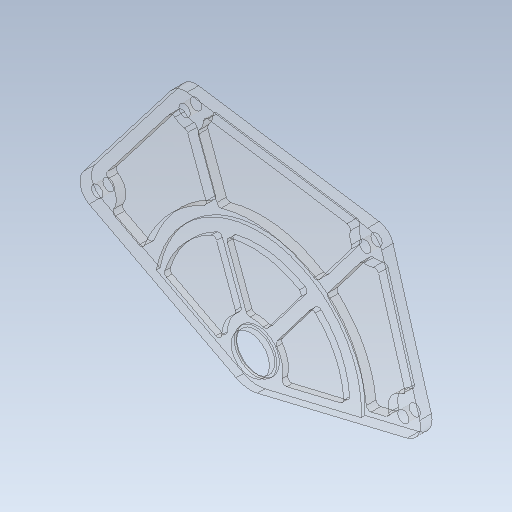
# Autodesk Inventor part: 後ろ脚外フレーム
Saved by Autodesk Inventor 2020 (Build 240168000, 168)
## iProperties
Created: 2019-09-18
Part Number: 後ろ脚外フレーム
Material: ポリカーボネート、クリア
Document SubType Name: Modeling
Designer: tanjihayato
Density: 1.2 g/cm^3
Appearance: ポリカーボネート - クリア
Mass: 5.9648 g
Surface Area: 89.9644 cm^2
Volume: 4.97067 cm^3
Author: tanjihayato
Autodesk Inventor part; units mm, degrees
ref_plane "YZ Plane" through (0, 0, 0) normal (1, 0, 0) x (0, 1, 0)
ref_plane "XZ Plane" through (0, 0, 0) normal (0, 1, 0) x (-1, 0, 0)
ref_plane "XY Plane" through (0, 0, 0) normal (0, 0, 1) x (1, 0, 0)
sketch "スケッチ1" plane through (0, 0, 0) normal (0, 0, 1) x (1, 0, 0)
  circle A0 centre (0, 0) radius 10.1 construction
  circle A1 centre (25.3202, -9.9362) radius 17.1 construction
  circle A2 centre (110.4743, -16.4118) radius 28.1 construction
  circle A3 centre (62.4131, -12.7569) radius 20.1 construction
  circle A4 centre (-21.6908, -16.4118) radius 17.1 construction
  circle A5 centre (-105.5257, -16.4118) radius 28.1 construction
  line L0 (-170.915, -81.4118) -> (490.0044, -81.4118)
  line L1 (-105.5257, -16.4118) -> (-21.6908, -16.4118) construction
  line L2 (110.4743, -16.4118) -> (25.3202, -9.9362) construction
  line L3 (110.4743, -16.4118) -> (104.1501, -0.632)
  line L4 (104.1501, -0.632) -> (95.5937, 20.7173) construction
  line L5 (95.5937, 20.7173) -> (70.4743, -10.4118) construction
  line L6 (70.4743, -10.4118) -> (110.4743, -16.4118) construction
  line L7 (-137.6819, 53.5882) -> (165.8186, 53.5882)
  line L8 (25.3202, -9.9362) -> (108.6869, 8.5882) construction
  line L9 (25.3202, -9.9362) -> (102.5386, -46.4118) construction
  line L10 (25.3202, -9.9362) -> (5.9362, 53.5882) construction
  line L11 (5.9362, 53.5882) -> (127.6431, 30.2622)
  line L12 (127.6431, 30.2622) -> (110.4743, -16.4118) construction
  line L13 (102.5386, -46.4118) -> (118.0681, 0.8329) construction
  line L14 (118.0681, 0.8329) -> (5.9362, 53.5882) construction
  line L15 (108.6869, 8.5882) -> (129.8583, 53.5882) construction
  line L16 (129.8583, 53.5882) -> (5.9362, 53.5882) construction
  line L17 (119.2726, 31.0882) -> (366.4441, 68.5882) construction
  line L18 (119.0587, 6.9252) -> (362.0213, 65.8249) construction
  line L19 (110.3034, -22.7894) -> (351.0624, 44.5537) construction
  line L20 (127.6431, 30.2622) -> (4.1927, 19.4617) construction
  circle A6 centre (80.4743, 23.124) radius 3 construction
  circle A7 centre (80.4743, 23.124) radius 1.5
  arc A8 (79.801, 27.5733) -> (76.162, 24.4099) centre (80.4743, 23.124) ccw
  circle A9 centre (70.4743, -10.4118) radius 1.5
  arc A10 (66.162, -9.1259) -> (69.4242, -14.7876) centre (70.4743, -10.4118) ccw
  circle A11 centre (150.4743, 0.5882) radius 1.5
  arc A12 (152.5623, -3.3981) -> (154.0408, 3.3323) centre (150.4743, 0.5882) ccw
  circle A13 centre (127.6431, 30.2622) radius 1.5
  arc A14 (131.2816, 32.9102) -> (126.9698, 34.7115) centre (127.6431, 30.2622) ccw
  circle A15 centre (110.4743, -16.4118) radius 5
  arc A16 (108.6075, -24.1909) -> (114.1862, -23.4986) centre (110.4743, -16.4118) ccw
  line L21 (76.162, 24.4099) -> (66.162, -9.1259)
  line L22 (69.4242, -14.7876) -> (108.6075, -24.1909)
  line L23 (114.1862, -23.4986) -> (152.5623, -3.3981)
  line L24 (154.0408, 3.3323) -> (131.2097, 33.0062)
  line L25 (126.9698, 34.7115) -> (79.801, 27.5733)
  circle A17 centre (-145.5257, 0.5882) radius 1.5
  arc A18 (-149.0922, 3.3323) -> (-147.6136, -3.3981) centre (-145.5257, 0.5882) ccw
  circle A19 centre (-105.5257, -16.4118) radius 5
  arc A20 (-109.2375, -23.4986) -> (-103.6588, -24.1909) centre (-105.5257, -16.4118) ccw
  circle A21 centre (-65.5257, -10.4118) radius 1.5
  arc A22 (-64.4756, -14.7876) -> (-61.2133, -9.1259) centre (-65.5257, -10.4118) ccw
  circle A23 centre (0, 0) radius 20.05 construction
  circle A24 centre (110.4743, -16.4118) radius 30.1 construction
  circle A25 centre (62.4131, -12.7569) radius 22.1 construction
  circle A26 centre (25.3202, -9.9362) radius 19.1 construction
  circle A27 centre (0, 0) radius 12.1 construction
  circle A28 centre (-21.6908, -16.4118) radius 19.1 construction
  circle A29 centre (-105.5257, -16.4118) radius 30.1 construction
  circle A30 centre (0, 0) radius 20.55 construction
  circle A31 centre (95.5937, 20.7173) radius 4.025 construction
  circle A32 centre (95.5937, 20.7173) radius 6.025 construction
  circle A33 centre (-75.5257, 23.124) radius 1.5
  arc A34 (-71.2133, 24.4099) -> (-74.8523, 27.5733) centre (-75.5257, 23.124) ccw
  circle A35 centre (-122.6945, 30.2622) radius 1.5
  arc A36 (-122.0212, 34.7115) -> (-126.261, 33.0062) centre (-122.6945, 30.2622) ccw
  line L26 (-126.261, 33.0062) -> (-149.0922, 3.3323)
  line L27 (-147.6136, -3.3981) -> (-109.2375, -23.4986)
  line L28 (-103.6588, -24.1909) -> (-64.4756, -14.7876)
  line L29 (-61.2133, -9.1259) -> (-71.2133, 24.4099)
  line L30 (-74.8523, 27.5733) -> (-122.0212, 34.7115)
  circle A37 centre (14, -17.4118) radius 2.2921 construction
  circle A38 centre (-14, -17.4118) radius 2.2921 construction
  circle A39 centre (-14, -17.4118) radius 14 construction
  circle A40 centre (14, -17.4118) radius 14 construction
  line L31 (-170.6512, -31.4118) -> (202.8656, -31.4118)
  line L32 (5.9362, 53.5882) -> (-38.6574, 35.6253) construction
  line L33 (5.9362, 53.5882) -> (-26.7676, 18.3503) construction
  circle A41 centre (5.9362, 53.5882) radius 1.5
  arc A42 (9.9603, 55.6024) -> (4.2549, 57.7623) centre (5.9362, 53.5882) ccw
  line L34 (-21.6908, -16.4118) -> (-99.9742, 13.5882) construction
  line L35 (-21.6908, -16.4118) -> (-101.7113, -41.4118) construction
  line L36 (9.9603, 55.6024) -> (33.1621, 9.2488)
  circle A43 centre (-47.0055, 32.2626) radius 1.5
  arc A44 (-48.6869, 36.4367) -> (-50.4404, 29.3554) centre (-47.0055, 32.2626) ccw
  line L37 (4.2549, 57.7623) -> (-48.6869, 36.4367)
  line L38 (-50.4404, 29.3554) -> (-38.6655, 15.4431)
  circle A45 centre (29.1381, 7.2346) radius 3 construction
  circle A46 centre (-84.8661, 5.2713) radius 4.5 construction
  circle A47 centre (-132.0174, -1.9813) radius 4.5 construction
  line L39 (-132.7015, 2.4664) -> (-85.5502, 9.719) construction
  arc A48 (28.3723, 2.8003) -> (33.1621, 9.2488) centre (29.1381, 7.2346) ccw
  arc A49 (-38.6655, 15.4431) -> (-35.9964, 13.9159) centre (-35.2306, 18.3503) ccw
  line L40 (-35.9964, 13.9159) -> (28.3723, 2.8003)
  circle A50 centre (-38.6574, 35.6253) radius 3 construction
  circle A51 centre (25.3202, -9.9362) radius 4.025 construction
  circle A52 centre (-21.6908, -16.4118) radius 4.025 construction
  circle A53 centre (-35.2306, 18.3503) radius 1.5
  circle A54 centre (29.1381, 7.2346) radius 1.5
  circle A55 centre (-57.813, 39.7705) radius 4.5 construction
  circle A56 centre (-99.304, 63.3152) radius 4.5 construction
  line L41 (5.9362, 53.5882) -> (-32.8159, 25.1361) construction
  circle A57 centre (-58.0056, -24.4791) radius 20.1 construction
  circle A58 centre (-58.0056, -24.4791) radius 22.1 construction
  line L42 (-53.3261, 39.4281) -> (-56.2797, 0.7243) construction
  circle A59 centre (-38.6574, 35.6253) radius 4.5
  dimension "d88" = 9
  dimension "d89" = 9
  dimension "d104" = 9
  dimension "d0" = 20.2
  dimension "d1" = 34.2
  dimension "d2" = 56.2
  dimension "d3" = 40.2
  dimension "d4" = 216
  dimension "d5" = 65
  dimension "d6" = 65
  dimension "d7" = 34.2
  dimension "d8" = 56.2
  dimension "d9" = 17
  dimension "d10" = 23
  dimension "d11" = 40
  dimension "d12" = 40
  dimension "d13" = 6
  dimension "d14" = 135
  dimension "d15" = 25
  dimension "d16" = 30
  dimension "d17" = 5
  dimension "d18" = 2
  dimension "d19" = 250
  dimension "d20" = 150
  dimension "d21" = 250
  dimension "d22" = 250
  dimension "d23" = 123.823
  dimension "d24" = 123.823
  dimension "d25" = 123.823
  dimension "d26" = 6
  dimension "d27" = 3
  dimension "d28" = 9
  dimension "d29" = 3
  dimension "d30" = 9
  dimension "d31" = 3
  dimension "d32" = 9
  dimension "d33" = 40
  dimension "d34" = 17
  dimension "d35" = 3
  dimension "d36" = 9
  dimension "d37" = 10
  dimension "d38" = 3
  dimension "d39" = 3
  dimension "d40" = 9
  dimension "d41" = 40
  dimension "d42" = 17
  dimension "d43" = 10
  dimension "d44" = 3
  dimension "d45" = 3
  dimension "d46" = 9
  dimension "d47" = 40
  dimension "d48" = 6
  dimension "d49" = 40.1
  dimension "d50" = 2
  dimension "d51" = 2
  dimension "d52" = 2
  dimension "d53" = 2
  dimension "d54" = 2
  dimension "d55" = 2
  dimension "d56" = 0.5
  dimension "d57" = 8.05
  dimension "d58" = 2
  dimension "d59" = 3
  dimension "d60" = 9
  dimension "d61" = 3
  dimension "d62" = 9
  dimension "d63" = 46.674
  constraints: 86 end point, 57 centre point, 39 tangent, 29 coincident, 29 point on circle, 11 equal length, 5 horizontal, 3 midpoint, 3 point on line, 2 equal radius, 1 collinear, 1 parallel, 1 perpendicular, 13 other
  measures "d0" diameter of A0
  measures "d1" diameter of A1
  measures "d2" diameter of A2
  measures "d3" diameter of A3
  measures "d4" distance of L1.start L2.start
  measures "d5" distance from line of L0 L2.start
  measures "d6" distance from line of L0 L1.start
  measures "d7" diameter of A4
  measures "d8" diameter of A5
  measures "d9" distance of L2.start L3.end
  measures "d10" distance of L3.end L4.end
  measures "d11" distance of L4.end L5.end
  measures "d12" horizontal distance of L5.end L2.start
  measures "d13" vertical distance of L5.end L2.start
  measures "d14" distance between parallel lines of L0 L7
  measures "d15" vertical distance of L2.start L8.end
  measures "d16" vertical distance of L9.end L2.start
  measures "d17" angle of L12 L15
  measures "d18" angle of L12 L13
  measures "d19" distance of L17.start L17.end
  measures "d20" distance from line of L0 L17.end
  measures "d21" distance of L18.start L18.end
  measures "d22" distance of L19.start L19.end
  measures "d23" angle of L15 L17
  measures "d24" angle of L12 L18
  measures "d25" angle of L13 L19
  measures "d26" diameter of A6
  measures "d27" diameter of A7
  measures "d28" diameter of A8
  measures "d29" diameter of A9
  measures "d30" diameter of A10
  measures "d31" diameter of A11
  measures "d32" diameter of A12
  measures "d33" horizontal distance of L2.start A11.centre
  measures "d34" vertical distance of L2.start A11.centre
  measures "d35" diameter of A13
  measures "d36" diameter of A14
  measures "d37" diameter of A15
  measures "d38" radial gap between concentric circles of A15 A16
  measures "d39" diameter of A17
  measures "d40" diameter of A18
  measures "d41" horizontal distance of L1.start A17.centre
  measures "d42" vertical distance of L1.start A18.centre
  measures "d43" diameter of A19
  measures "d44" radial gap between concentric circles of A19 A20
  measures "d45" diameter of A21
  measures "d46" diameter of A22
  measures "d47" horizontal distance of L1.start A21.centre
  measures "d48" vertical distance of L1.start A21.centre
  measures "d49" diameter of A23
  measures "d50" radial gap between concentric circles of A2 A24
  measures "d51" radial gap between concentric circles of A3 A25
  measures "d52" radial gap between concentric circles of A1 A26
  measures "d53" radial gap between concentric circles of A0 A27
  measures "d54" radial gap between concentric circles of A4 A28
  measures "d55" radial gap between concentric circles of A5 A29
  measures "d56" radial gap between concentric circles of A23 A30
  measures "d57" diameter of A31
  measures "d58" radial gap between concentric circles of A31 A32
  measures "d59" diameter of A33
  measures "d60" diameter of A34
  measures "d61" diameter of A35
  measures "d62" diameter of A36
  measures "d63" vertical distance of L2.start L11.end
extrude "押し出し1" add sketch "スケッチ1" along normal blind 3 contours L26 A36 L30 A34 L29 A22 L28 A20 L27 A18
sketch "スケッチ2" plane through (0, 0, 0) normal (0, 0, -1) x (-1, 0, 0)
  circle A0 centre (105.5257, -16.4118) radius 5 projected
  circle A1 centre (122.6945, 30.2622) radius 1.5 projected
  circle A2 centre (75.5257, 23.124) radius 1.5 projected
  circle A3 centre (65.5257, -10.4118) radius 1.5 projected
  circle A4 centre (145.5257, 0.5882) radius 1.5 projected
  line L0 (149.0922, 3.3323) -> (126.261, 33.0062) projected
  arc A5 (126.261, 33.0062) -> (122.0212, 34.7115) centre (122.6945, 30.2622) ccw projected
  line L1 (122.0212, 34.7115) -> (74.8523, 27.5733) projected
  arc A6 (74.8523, 27.5733) -> (71.2133, 24.4099) centre (75.5257, 23.124) ccw projected
  line L2 (71.2133, 24.4099) -> (61.2133, -9.1259) projected
  arc A7 (61.2133, -9.1259) -> (64.4756, -14.7876) centre (65.5257, -10.4118) ccw projected
  line L3 (64.4756, -14.7876) -> (103.6588, -24.1909) projected
  arc A8 (103.6588, -24.1909) -> (109.2375, -23.4986) centre (105.5257, -16.4118) ccw projected
  line L4 (109.2375, -23.4986) -> (147.6136, -3.3981) projected
  arc A9 (147.6136, -3.3981) -> (149.0922, 3.3323) centre (145.5257, 0.5882) ccw projected
  line L5 (75.3012, 24.6071) -> (122.47, 31.7453)
  arc A10 (123.8833, 31.1769) -> (122.47, 31.7453) centre (122.6945, 30.2622) ccw
  line L6 (123.8833, 31.1769) -> (146.7145, 1.5029)
  arc A11 (146.2216, -0.7406) -> (146.7145, 1.5029) centre (145.5257, 0.5882) ccw
  line L7 (146.2216, -0.7406) -> (107.8456, -20.841)
  arc A12 (104.3589, -21.2738) -> (107.8456, -20.841) centre (105.5257, -16.4118) ccw
  line L8 (104.3589, -21.2738) -> (65.1756, -11.8704)
  arc A13 (64.0882, -9.9832) -> (65.1756, -11.8704) centre (65.5257, -10.4118) ccw
  line L9 (64.0882, -9.9832) -> (74.0882, 23.5526)
  arc A14 (75.3012, 24.6071) -> (74.0882, 23.5526) centre (75.5257, 23.124) ccw
  circle A15 centre (75.5257, 23.124) radius 4.5
  circle A16 centre (65.5257, -10.4118) radius 4.5
  circle A17 centre (105.5257, -16.4118) radius 8
  circle A18 centre (145.5257, 0.5882) radius 4.5
  circle A19 centre (122.6945, 30.2622) radius 4.5
  arc A20 (132.0813, -11.5335) -> (78.5832, -18.1732) centre (105.5257, -16.4118) ccw
  circle A21 centre (105.5257, -16.4118) radius 5.6
  line L10 (105.5257, -16.4118) -> (75.5257, 23.124) construction
  line L11 (106.7206, -15.5051) -> (76.7206, 24.0307)
  line L12 (74.3307, 22.2173) -> (104.3307, -17.3185)
  arc A22 (104.3307, -17.3185) -> (106.7206, -15.5051) centre (105.5257, -16.4118) ccw
  arc A23 (76.7206, 24.0307) -> (74.3307, 22.2173) centre (75.5257, 23.124) ccw
  line L13 (105.5257, -16.4118) -> (122.6945, 30.2622) construction
  line L14 (106.9334, -16.9296) -> (124.1023, 29.7443)
  line L15 (121.2867, 30.78) -> (104.1179, -15.894)
  arc A24 (104.1179, -15.894) -> (106.9334, -16.9296) centre (105.5257, -16.4118) ccw
  arc A25 (124.1023, 29.7443) -> (121.2867, 30.78) centre (122.6945, 30.2622) ccw
  arc A26 (134.8505, -10.0831) -> (75.5434, -17.4437) centre (105.5257, -16.4118) ccw
  arc A27 (129.2819, -12.9998) -> (81.6561, -18.9106) centre (105.5257, -16.4118) ccw
  point P0 (0, 0)
  point P1 (90.5257, 3.3561)
  point P2 (114.1101, 6.9252)
  dimension "d120" = 3
  dimension "d121" = 3
  dimension "d122" = 3
  dimension "d123" = 3
  dimension "d124" = 3
  dimension "d125" = 3
  dimension "d126" = 54
  dimension "d127" = 0.6
  dimension "d128" = 3
  dimension "d129" = 3
  dimension "d130" = 3
  dimension "d131" = 3
  constraints: 26 end point, 24 point on circle, 18 centre point, 8 tangent, 6 point on line, 2 midpoint, 2 parallel, 1 coincident, 9 other
  measures "d120" distance between parallel lines of L1 L5
  measures "d121" radial gap between concentric circles of A2 A15
  measures "d122" radial gap between concentric circles of A3 A16
  measures "d123" radial gap between concentric circles of A0 A17
  measures "d124" radial gap between concentric circles of A4 A18
  measures "d125" radial gap between concentric circles of A1 A19
  measures "d126" diameter of A20
  measures "d127" radial gap between concentric circles of A0 A21
  measures "d128" diameter of A23
  measures "d129" diameter of A25
  measures "d130" radial gap between concentric circles of A20 A26
  measures "d131" radial gap between concentric circles of A20 A27
extrude "押し出し2" cut sketch "スケッチ2" against normal blind 2.5 contours L8 A21 L12 A0 | A0 L14 A21 L7 | L8 A17 L12 A21 | A21 L14 A17 L7 | L11 A21 L15 A0 | L8 A27 L12 A17 | A17 L14 A27 L7 | L11 A17 L15 A21 | L8 A20 L12 A27 | A27 L14 A20 L7 | L11 A27 L15 A17 | L8 A26 L12 A20 | A20 L14 A26 L7 | L11 A20 L15 A27 | L8 A16 L9 A15 L12 A26 | A26 L14 A19 L6 A18 L7 | L11 A26 L15 A20 | L8 A3 L9 A16 | A18 L6 A4 L7 | L11 A15 L5 A19 L15 A26 | A15 L9 A2 L12 | L14 A1 L6 A19 | L11 A2 L5 A15 | A19 L5 A1 L15
extrude "押し出し3" add sketch "スケッチ2" against normal blind 3 contours L8 A21 L12 A0 | A0 L7 A21 L8 | A0 L14 A21 L7 | L12 A21 L11 A0 | A21 L7 A17 A8 L8 | L8 A17 L12 A21 | A21 L14 A17 L7 | L11 A21 L15 A0 | L12 A17 L11 A21 | A0 L15 A21 L14 | L11 A17 L15 A21 | A27 L3 A20 L8 | L8 A20 L12 A27 | A21 L15 A17 L14 | A27 L14 A20 L7 | L7 A20 L4 A27 | L12 A20 L11 A27 | A20 L3 A26 L8 | L8 A26 L12 A20 | A20 L14 A26 L7 | L7 A26 L4 A20 | A27 L15 A20 L14 | L11 A20 L15 A27 | L12 A26 L11 A20 | A20 L15 A26 L14 | L11 A26 L15 A20 | A16 A7 L9 A3 L8 | L8 A3 L9 A16 | A18 L6 A4 L7 | L7 A4 L6 A18 A9 | L12 A2 L11 A15 | A15 L9 A2 L12 | L14 A1 L6 A19 | A19 L15 A1 L14 | L11 A2 L5 A15 | A15 A6 L5 A2 L9 | L6 A1 L5 A19 A5 | A19 L5 A1 L15
extrude "押し出し4" cut sketch "スケッチ2" against normal blind 1 contours L8 A21 L12 A0 | A0 L7 A21 L8 | A0 L14 A21 L7 | L12 A21 L11 A0 | A21 L7 A17 A8 L8 | L8 A17 L12 A21 | A21 L14 A17 L7 | L11 A21 L15 A0 | L12 A17 L11 A21 | A17 L3 A27 L8 | L8 A27 L12 A17 | A0 L15 A21 L14 | A17 L14 A27 L7 | L7 A27 L4 A17 | L11 A17 L15 A21 | L12 A27 L11 A17 | A27 L3 A20 L8 | L8 A20 L12 A27 | A21 L15 A17 L14 | A27 L14 A20 L7 | L7 A20 L4 A27 | L11 A27 L15 A17 | L12 A20 L11 A27 | A17 L15 A27 L14 | A27 L15 A20 L14 | L11 A20 L15 A27
extrude "押し出し5" cut sketch "スケッチ2" against normal blind 1.6 contours L8 A21 L12 A0 | A0 L7 A21 L8 | A0 L14 A21 L7 | L12 A21 L11 A0 | L11 A21 L15 A0 | A0 L15 A21 L14
fillet "フィレット1" radius 1 30 edges at (-65.3006, -5.9174, 1.25) (-69.3011, -12.8604, 1.25) (-75.5952, -14.3709, 1.25) (-81.5336, -15.796, 1.75) (-98.2863, -19.8164, 1.75) (-99.5807, -11.0586, 1.75) (-89.8516, 1.763, 1.75) (-92.2414, 3.5764, 1.75) (-101.9705, -9.2451, 1.75) (-106.8307, -8.519, 1.75) (-109.6463, -9.5547, 1.75) (-113.3777, -17.9434, 1.75) (-128.6393, -9.9498, 1.75) (-115.2028, 5.5508, 1.75) (-112.3872, 6.5864, 1.75) (-134.0492, -7.1162, 1.25) (-117.2774, 11.1907, 1.25) (-114.4618, 12.2264, 1.25) (-122.6376, 25.7625, 1.25) (-126.4705, 27.8143, 1.25) (-144.1274, 4.8654, 1.25) (-142.4633, -2.7091, 1.25) (-119.822, 26.7982, 1.25) (-118.2752, 31.1105, 1.25) (-79.4961, 25.2419, 1.25) (-79.2852, 20.6509, 1.25) (-88.6089, 8.3636, 1.25) (-86.219, 6.5502, 1.25) (-76.8953, 18.8375, 1.25) (-72.8759, 19.4869, 1.25)
equation "\"d7\" = d1"
equation "\"d8\" = d2"
equation "\"d24\" = d23"
equation "\"d25\" = d23"
